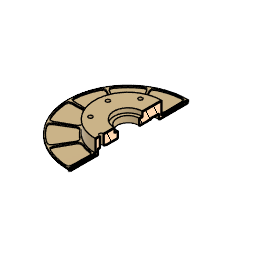
Brodie Stator Bottom (Autodesk Fusion 360 design; units mm, degrees)
Autodesk Fusion 360 part; units mm, degrees
sketch "Sketch1" plane through (0, 0, 0) normal (0, 0, 1) x (1, 0, 0)
  circle A0 centre (0, 0) radius 26
  circle A1 centre (0, 0) radius 47
  constraint coincident A0.centre A1.centre
  constraint concentric A0 A1
extrude "Extrude1" add sketch "Sketch1" along normal blind 2 contours A0 | A1
sketch "Sketch2" plane through (0, 0, 2) normal (0, 0, 1) x (-1, 0, 0)
  circle A0 centre (0, 0) radius 47
  circle A1 centre (0, 0) radius 26
  constraint coincident A0.centre A1.centre
extrude "Extrude2" add sketch "Sketch2" along normal blind 10 contours A1
sketch "Sketch3" plane through (0, 0, 0) normal (0, 0, -1) x (1, 0, 0)
  circle A0 centre (0, 0) radius 47
  circle A1 centre (0, 0) radius 24
  constraint coincident A0.centre A1.centre
extrude "Extrude3" cut sketch "Sketch3" against normal blind 3.5 contours A1
sketch "Sketch4" plane through (0, 0, 12) normal (0, 0, 1) x (-1, 0, 0)
  circle A0 centre (0, 0) radius 26
  circle A1 centre (0, 0) radius 8.5
  dimension "d7" = 17
  constraint concentric A0 A1
  measures "d7" diameter of A1
extrude "Extrude4" cut sketch "Sketch4" against normal blind 10 contours A1
sketch "Sketch5" plane through (0, 0, 12) normal (0, 0, 1) x (-1, 0, 0)
  circle A0 centre (0, 0) radius 8.5
  circle A1 centre (0, 0) radius 26
  circle A2 centre (0, 0) radius 11
  constraint coincident A0.centre A1.centre
extrude "Extrude5" cut sketch "Sketch5" against normal blind 3.5 contours A2
sketch "Sketch6" plane through (0, 0, 3.5) normal (0, 0, -1) x (1, 0, 0)
  circle A0 centre (0, 0) radius 8.5
  circle A1 centre (0, 0) radius 24
  circle A2 centre (0, 0) radius 18
  dimension "d12" = 36
  constraint concentric A0 A2
  measures "d12" diameter of A2
extrude "Extrude6" cut sketch "Sketch6" against normal blind 1.5 contours A1
fillet "Fillet1" radius 1 1 edges at (-43.8194, -16.9959, 0)
sketch "Sketch7" plane through (0, 0, 5) normal (0, 0, -1) x (1, 0, 0)
  circle A0 centre (0, 0) radius 18
  circle A1 centre (0, 0) radius 24
  circle A2 centre (0, 21) radius 1.5
  circle A3 centre (0, 21) radius 2.7
  circle A4 centre (-16.4185, 13.0933) radius 2.7
  circle A5 centre (-16.4185, 13.0933) radius 1.5
  circle A6 centre (-20.4735, -4.6729) radius 2.7
  circle A7 centre (-20.4735, -4.6729) radius 1.5
  circle A8 centre (-9.1116, -18.9203) radius 2.7
  circle A9 centre (-9.1116, -18.9203) radius 1.5
  circle A10 centre (9.1116, -18.9203) radius 2.7
  circle A11 centre (9.1116, -18.9203) radius 1.5
  circle A12 centre (20.4735, -4.6729) radius 2.7
  circle A13 centre (20.4735, -4.6729) radius 1.5
  circle A14 centre (16.4185, 13.0933) radius 2.7
  circle A15 centre (16.4185, 13.0933) radius 1.5
  dimension "d17" = 5.4
  dimension "d19" = 360
  constraint concentric A2 A3
  measures "d17" diameter of A3
extrude "Extrude7" cut sketch "Sketch7" against normal blind 10 contours A2 | A5 | A7 | A9 | A11 | A13 | A15
sketch "Sketch8" plane through (0, 0, 2) normal (0, 0, 1) x (-1, 0, 0)
  circle A0 centre (0, 0) radius 26
  circle A1 centre (0, 0) radius 47
  line L0 (-0.5209, -29.8451) -> (-0.7486, -42.8887)
  arc A2 (-19.44, -41.6904) -> (-4.0097, -45.8249) centre (0, 0) ccw
  line L1 (-14.4714, -26.1071) -> (-20.796, -37.517)
  arc A3 (-10.6628, -24.8053) -> (-3.1684, -26.8134) centre (0, 0) ccw
  arc A4 (-0.5209, -29.8451) -> (-3.1684, -26.8134) centre (-3.5205, -29.7927) ccw
  arc A5 (-10.6628, -24.8053) -> (-14.4714, -26.1071) centre (-11.8475, -27.5615) ccw
  arc A6 (4.0097, -45.8249) -> (19.44, -41.6904) centre (0, 0) ccw
  arc A7 (0.7486, -42.8887) -> (4.0097, -45.8249) centre (3.7482, -42.8363) ccw
  line L2 (0.5209, -29.8451) -> (0.7486, -42.8887)
  arc A8 (3.1684, -26.8134) -> (0.5209, -29.8451) centre (3.5205, -29.7927) ccw
  arc A9 (3.1684, -26.8134) -> (10.6628, -24.8053) centre (0, 0) ccw
  arc A10 (14.4714, -26.1071) -> (10.6628, -24.8053) centre (11.8475, -27.5615) ccw
  line L3 (14.4714, -26.1071) -> (20.796, -37.517)
  arc A11 (19.44, -41.6904) -> (20.796, -37.517) centre (18.1722, -38.9714) ccw
  arc A12 (26.3849, -37.6807) -> (37.6807, -26.3849) centre (0, 0) ccw
  arc A13 (22.0927, -36.7684) -> (26.3849, -37.6807) centre (24.6642, -35.2233) ccw
  line L4 (15.3737, -25.5861) -> (22.0927, -36.7684)
  arc A14 (16.1507, -21.6369) -> (15.3737, -25.5861) centre (17.9452, -24.041) ccw
  arc A15 (16.1507, -21.6369) -> (21.6369, -16.1507) centre (0, 0) ccw
  arc A16 (25.5861, -15.3737) -> (21.6369, -16.1507) centre (24.041, -17.9452) ccw
  line L5 (25.5861, -15.3737) -> (36.7684, -22.0927)
  arc A17 (37.6807, -26.3849) -> (36.7684, -22.0927) centre (35.2233, -24.6642) ccw
  arc A18 (41.6904, -19.44) -> (45.8249, -4.0097) centre (0, 0) ccw
  arc A19 (37.517, -20.796) -> (41.6904, -19.44) centre (38.9714, -18.1722) ccw
  line L6 (26.1071, -14.4714) -> (37.517, -20.796)
  arc A20 (24.8053, -10.6628) -> (26.1071, -14.4714) centre (27.5615, -11.8475) ccw
  arc A21 (24.8053, -10.6628) -> (26.8134, -3.1684) centre (0, 0) ccw
  arc A22 (29.8451, -0.5209) -> (26.8134, -3.1684) centre (29.7927, -3.5205) ccw
  line L7 (29.8451, -0.5209) -> (42.8887, -0.7486)
  arc A23 (45.8249, -4.0097) -> (42.8887, -0.7486) centre (42.8363, -3.7482) ccw
  arc A24 (45.8249, 4.0097) -> (41.6904, 19.44) centre (0, 0) ccw
  arc A25 (42.8887, 0.7486) -> (45.8249, 4.0097) centre (42.8363, 3.7482) ccw
  line L8 (29.8451, 0.5209) -> (42.8887, 0.7486)
  arc A26 (26.8134, 3.1684) -> (29.8451, 0.5209) centre (29.7927, 3.5205) ccw
  arc A27 (26.8134, 3.1684) -> (24.8053, 10.6628) centre (0, 0) ccw
  arc A28 (26.1071, 14.4714) -> (24.8053, 10.6628) centre (27.5615, 11.8475) ccw
  line L9 (26.1071, 14.4714) -> (37.517, 20.796)
  arc A29 (41.6904, 19.44) -> (37.517, 20.796) centre (38.9714, 18.1722) ccw
  arc A30 (37.6807, 26.3849) -> (26.3849, 37.6807) centre (0, 0) ccw
  arc A31 (36.7684, 22.0927) -> (37.6807, 26.3849) centre (35.2233, 24.6642) ccw
  line L10 (25.5861, 15.3737) -> (36.7684, 22.0927)
  arc A32 (21.6369, 16.1507) -> (25.5861, 15.3737) centre (24.041, 17.9452) ccw
  arc A33 (21.6369, 16.1507) -> (16.1507, 21.6369) centre (0, 0) ccw
  arc A34 (15.3737, 25.5861) -> (16.1507, 21.6369) centre (17.9452, 24.041) ccw
  line L11 (15.3737, 25.5861) -> (22.0927, 36.7684)
  arc A35 (26.3849, 37.6807) -> (22.0927, 36.7684) centre (24.6642, 35.2233) ccw
  arc A36 (19.44, 41.6904) -> (4.0097, 45.8249) centre (0, 0) ccw
  arc A37 (20.796, 37.517) -> (19.44, 41.6904) centre (18.1722, 38.9714) ccw
  line L12 (14.4714, 26.1071) -> (20.796, 37.517)
  arc A38 (10.6628, 24.8053) -> (14.4714, 26.1071) centre (11.8475, 27.5615) ccw
  arc A39 (10.6628, 24.8053) -> (3.1684, 26.8134) centre (0, 0) ccw
  arc A40 (0.5209, 29.8451) -> (3.1684, 26.8134) centre (3.5205, 29.7927) ccw
  line L13 (0.5209, 29.8451) -> (0.7486, 42.8887)
  arc A41 (4.0097, 45.8249) -> (0.7486, 42.8887) centre (3.7482, 42.8363) ccw
  arc A42 (-4.0097, 45.8249) -> (-19.44, 41.6904) centre (0, 0) ccw
  arc A43 (-0.7486, 42.8887) -> (-4.0097, 45.8249) centre (-3.7482, 42.8363) ccw
  line L14 (-0.5209, 29.8451) -> (-0.7486, 42.8887)
  arc A44 (-3.1684, 26.8134) -> (-0.5209, 29.8451) centre (-3.5205, 29.7927) ccw
  arc A45 (-3.1684, 26.8134) -> (-10.6628, 24.8053) centre (0, 0) ccw
  arc A46 (-14.4714, 26.1071) -> (-10.6628, 24.8053) centre (-11.8475, 27.5615) ccw
  line L15 (-14.4714, 26.1071) -> (-20.796, 37.517)
  arc A47 (-19.44, 41.6904) -> (-20.796, 37.517) centre (-18.1722, 38.9714) ccw
  arc A48 (-26.3849, 37.6807) -> (-37.6807, 26.3849) centre (0, 0) ccw
  arc A49 (-22.0927, 36.7684) -> (-26.3849, 37.6807) centre (-24.6642, 35.2233) ccw
  line L16 (-15.3737, 25.5861) -> (-22.0927, 36.7684)
  arc A50 (-16.1507, 21.6369) -> (-15.3737, 25.5861) centre (-17.9452, 24.041) ccw
  arc A51 (-16.1507, 21.6369) -> (-21.6369, 16.1507) centre (0, 0) ccw
  arc A52 (-25.5861, 15.3737) -> (-21.6369, 16.1507) centre (-24.041, 17.9452) ccw
  line L17 (-25.5861, 15.3737) -> (-36.7684, 22.0927)
  arc A53 (-37.6807, 26.3849) -> (-36.7684, 22.0927) centre (-35.2233, 24.6642) ccw
  arc A54 (-41.6904, 19.44) -> (-45.8249, 4.0097) centre (0, 0) ccw
  arc A55 (-37.517, 20.796) -> (-41.6904, 19.44) centre (-38.9714, 18.1722) ccw
  line L18 (-26.1071, 14.4714) -> (-37.517, 20.796)
  arc A56 (-24.8053, 10.6628) -> (-26.1071, 14.4714) centre (-27.5615, 11.8475) ccw
  arc A57 (-24.8053, 10.6628) -> (-26.8134, 3.1684) centre (0, 0) ccw
  arc A58 (-29.8451, 0.5209) -> (-26.8134, 3.1684) centre (-29.7927, 3.5205) ccw
  line L19 (-29.8451, 0.5209) -> (-42.8887, 0.7486)
  arc A59 (-45.8249, 4.0097) -> (-42.8887, 0.7486) centre (-42.8363, 3.7482) ccw
  arc A60 (-45.8249, -4.0097) -> (-41.6904, -19.44) centre (0, 0) ccw
  arc A61 (-42.8887, -0.7486) -> (-45.8249, -4.0097) centre (-42.8363, -3.7482) ccw
  line L20 (-29.8451, -0.5209) -> (-42.8887, -0.7486)
  arc A62 (-26.8134, -3.1684) -> (-29.8451, -0.5209) centre (-29.7927, -3.5205) ccw
  arc A63 (-26.8134, -3.1684) -> (-24.8053, -10.6628) centre (0, 0) ccw
  arc A64 (-26.1071, -14.4714) -> (-24.8053, -10.6628) centre (-27.5615, -11.8475) ccw
  line L21 (-26.1071, -14.4714) -> (-37.517, -20.796)
  arc A65 (-41.6904, -19.44) -> (-37.517, -20.796) centre (-38.9714, -18.1722) ccw
  arc A66 (-37.6807, -26.3849) -> (-26.3849, -37.6807) centre (0, 0) ccw
  arc A67 (-36.7684, -22.0927) -> (-37.6807, -26.3849) centre (-35.2233, -24.6642) ccw
  line L22 (-25.5861, -15.3737) -> (-36.7684, -22.0927)
  arc A68 (-21.6369, -16.1507) -> (-25.5861, -15.3737) centre (-24.041, -17.9452) ccw
  arc A69 (-21.6369, -16.1507) -> (-16.1507, -21.6369) centre (0, 0) ccw
  arc A70 (-15.3737, -25.5861) -> (-16.1507, -21.6369) centre (-17.9452, -24.041) ccw
  line L23 (-15.3737, -25.5861) -> (-22.0927, -36.7684)
  arc A71 (-20.796, -37.517) -> (-21.1397, -39.4118) centre (-18.1722, -38.9714) ccw
  arc A72 (-20.8317, -40.3595) -> (-19.44, -41.6904) centre (-18.1722, -38.9714) ccw
  arc A73 (-21.1397, -39.4118) -> (-20.8317, -40.3595) centre (-21.0253, -39.8985) ccw
  arc A74 (-4.0097, -45.8249) -> (-2.139, -45.3682) centre (-3.7482, -42.8363) ccw
  arc A75 (-1.3984, -44.7014) -> (-0.7486, -42.8887) centre (-3.7482, -42.8363) ccw
  arc A76 (-2.139, -45.3682) -> (-1.3984, -44.7014) centre (-1.7408, -45.0658) ccw
  arc A77 (1.3984, -44.7014) -> (2.139, -45.3682) centre (1.7408, -45.0658) ccw
  arc A78 (20.8317, -40.3595) -> (21.1397, -39.4118) centre (21.0253, -39.8985) ccw
  arc A79 (23.5617, -38.0134) -> (24.5365, -38.2205) centre (24.0405, -38.1577) ccw
  arc A80 (38.2205, -24.5365) -> (38.0134, -23.5617) centre (38.1577, -24.0405) ccw
  arc A81 (39.4118, -21.1397) -> (40.3595, -20.8317) centre (39.8985, -21.0253) ccw
  arc A82 (45.3682, -2.139) -> (44.7014, -1.3984) centre (45.0658, -1.7408) ccw
  arc A83 (44.7014, 1.3984) -> (45.3682, 2.139) centre (45.0658, 1.7408) ccw
  arc A84 (40.3595, 20.8317) -> (39.4118, 21.1397) centre (39.8985, 21.0253) ccw
  arc A85 (38.0134, 23.5617) -> (38.2205, 24.5365) centre (38.1577, 24.0405) ccw
  arc A86 (24.5365, 38.2205) -> (23.5617, 38.0134) centre (24.0405, 38.1577) ccw
  arc A87 (21.1397, 39.4118) -> (20.8317, 40.3595) centre (21.0253, 39.8985) ccw
  arc A88 (2.139, 45.3682) -> (1.3984, 44.7014) centre (1.7408, 45.0658) ccw
  arc A89 (-1.3984, 44.7014) -> (-2.139, 45.3682) centre (-1.7408, 45.0658) ccw
  arc A90 (-20.8317, 40.3595) -> (-21.1397, 39.4118) centre (-21.0253, 39.8985) ccw
  arc A91 (-23.5617, 38.0134) -> (-24.5365, 38.2205) centre (-24.0405, 38.1577) ccw
  arc A92 (-38.2205, 24.5365) -> (-38.0134, 23.5617) centre (-38.1577, 24.0405) ccw
  arc A93 (-39.4118, 21.1397) -> (-40.3595, 20.8317) centre (-39.8985, 21.0253) ccw
  arc A94 (-45.3682, 2.139) -> (-44.7014, 1.3984) centre (-45.0658, 1.7408) ccw
  arc A95 (-44.7014, -1.3984) -> (-45.3682, -2.139) centre (-45.0658, -1.7408) ccw
  arc A96 (-40.3595, -20.8317) -> (-39.4118, -21.1397) centre (-39.8985, -21.0253) ccw
  arc A97 (-38.0134, -23.5617) -> (-38.2205, -24.5365) centre (-38.1577, -24.0405) ccw
  arc A98 (-24.5365, -38.2205) -> (-23.5617, -38.0134) centre (-24.0405, -38.1577) ccw
  arc A99 (-26.3849, -37.6807) -> (-24.5365, -38.2205) centre (-24.6642, -35.2233) ccw
  arc A100 (-23.5617, -38.0134) -> (-22.0927, -36.7684) centre (-24.6642, -35.2233) ccw
  point P0 (-0.8028, -45.993)
  dimension "d28" = 3
  dimension "d29" = 3
  dimension "d30" = 3
  dimension "d31" = 3
  dimension "d33" = 360
  dimension "d34" = 1
  dimension "d35" = 1
  dimension "d37" = 360
  constraint coincident A0.centre A1.centre
  constraint coincident P0 L0
  constraint tangent L0 A75
  constraint tangent A2 A74
  constraint tangent L1 A71
  constraint tangent A2 A72
  constraint tangent A3 A4
  constraint tangent L0 A4
  constraint tangent A3 A5
  constraint tangent L1 A5
  constraint concentric A71 A72
  constraint concentric A74 A75
  constraint concentric A99 A100
  constraint coincident A76.centre A75
  constraint coincident A73.centre A72
  measures "d28" radius of A74
  measures "d29" radius of A71
  measures "d30" radius of A4
  measures "d31" radius of A5
  measures "d34" diameter of A76
  measures "d35" diameter of A73
extrude "Extrude8" cut sketch "Sketch8" against normal blind 1 contours L0 A2 L1 A3 A4 A5 A71 A72 A73 A74 A75 A76
extrude "Extrude9" cut sketch "Sketch8" against normal blind 1 contours A6 A7 L2 A8 A9 A10 L3 A11 | A11 A78 | A12 A13 L4 A14 A15 A16 L5 A17 | A13 A79 | A17 A80 | A18 A19 L6 A20 A21 A22 L7 A23 | A19 A81 | A23 A82 | A24 A25 L8 A26 A27 A28 L9 A29 | A25 A83 | A29 A84 | A30 A31 L10 A32 A33 A34 L11 A35 | A31 A85 | A35 A86 | A36 A37 L12 A38 A39 A40 L13 A41 | A37 A87 | A41 A88 | A42 A43 L14 A44 A45 A46 L15 A47 | A43 A89 | A47 A90
extrude "Extrude10" cut sketch "Sketch8" against normal blind 1 contours A7 A77 | A48 A49 L16 A50 A51 A52 L17 A53 | A49 A91 | A53 A92 | A54 A55 L18 A56 A57 A58 L19 A59 | A55 A93 | A59 A94 | A60 A61 L20 A62 A63 A64 L21 A65 | A61 A95 | A65 A96 | A66 A67 L22 A68 A69 A70 L23 A98 A99 A100 | A67 A97
extrude "Extrude11" add 1 faces at (-15.2506, 15.7771, 5) along direction (0, 0, -1) blind 1
